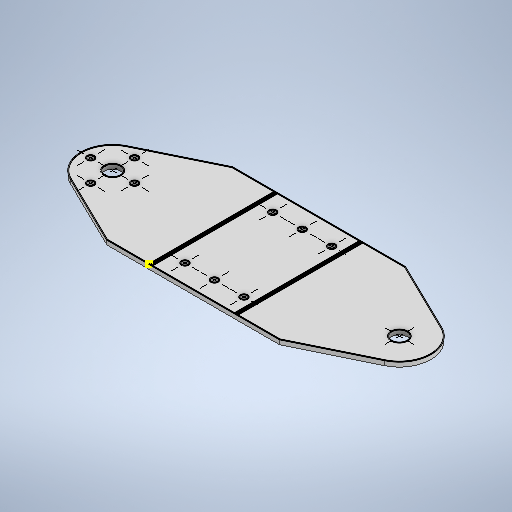
# Autodesk Inventor part: CAM_axis_6_supplement_frame
Saved by Autodesk Inventor 2025.2 (Build 292293000, 293)
## iProperties
Created: 2025-08-09
Part Number: CAM_axis_6_supplement_frame
Material: Generic
Document SubType Name: Modeling
Designer: User
Density: 1 g/cm^3
Appearance: Default
Author: User
Autodesk Inventor part; units mm, degrees
ref_plane "YZ Plane" through (0, 0, 0) normal (1, 0, 0) x (0, 1, 0)
ref_plane "XZ Plane" through (0, 0, 0) normal (0, 1, 0) x (-1, 0, 0)
ref_plane "XY Plane" through (0, 0, 0) normal (0, 0, 1) x (1, 0, 0)
sketch "Sketch1" plane through (0, 0, 0) normal (0, 1, 0) x (-1, 0, 0)
  line L0 (-0.4496, -40) -> (-0.4496, 0)
  line L1 (-27.6589, 0) -> (-27.6589, -40)
  circle A0 centre (-5.3993, -34) radius 1.05
  circle A1 centre (-14.8043, -34) radius 1.05
  circle A2 centre (-24.2093, -34) radius 1.05
  circle A3 centre (-24.2093, -6) radius 1.05
  circle A4 centre (-14.8043, -6) radius 1.05
  circle A5 centre (-5.3993, -6) radius 1.05
  circle A6 centre (-59.7986, -20) radius 2.55
  circle A7 centre (31.69, -20) radius 2.6
  circle A8 centre (24.69, -20) radius 1.05
  circle A9 centre (31.69, -13) radius 1.05
  circle A10 centre (31.69, -27) radius 1.05
  circle A11 centre (38.69, -20) radius 1.05
  line L2 (36.0744, -11.0124) -> (13.5, 0)
  line L3 (-41.6086, 0) -> (-64.183, -11.0124)
  line L4 (13.5, -40) -> (36.0744, -28.9876)
  line L5 (-64.183, -28.9876) -> (-41.6086, -40)
  arc A12 (36.0744, -28.9876) -> (36.0744, -11.0124) centre (31.69, -20) ccw
  arc A13 (-64.183, -11.0124) -> (-64.183, -28.9876) centre (-59.7986, -20) ccw
  line L6 (-41.6086, 0) -> (13.5, 0)
  line L7 (13.5, -40) -> (-41.6086, -40)
  line L8 (-28.1086, -40) -> (-28.1086, 0)
  line L9 (-27.2093, 0) -> (-27.2093, -40)
  line L10 (-0.8993, -40) -> (-0.8993, 0)
  line L11 (0, 0) -> (0, -40)
  constraints: 24 end point, 14 centre point, 12 point on line, 10 equal radius, 7 parallel, 6 vertical, 4 point on circle, 4 tangent, 2 horizontal, 2 perpendicular, 51 other
extrude "Extrusion1" add sketch "Sketch1" against normal blind 1.5
body "Solid1"
